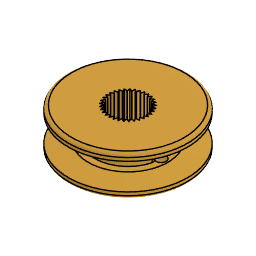
Spool_v4 (Autodesk Fusion 360 design; units mm, degrees)
Autodesk Fusion 360 part; units mm, degrees
sketch "Sketch1" plane through (0, 0, 0) normal (0, 0, 1) x (1, 0, 0)
  line L0 (-0.0246, -2.4999) -> (0.1607, -2.8207)
  line L1 (0.1607, -2.8207) -> (0.3083, -2.4809)
  arc A0 (0.3083, -2.4809) -> (0.449, -2.4594) centre (0, 0) ccw
  line L2 (0.449, -2.4594) -> (0.6916, -2.7393)
  line L3 (0.6916, -2.7393) -> (0.7722, -2.3777)
  arc A1 (0.7722, -2.3777) -> (0.9063, -2.3299) centre (0, 0) ccw
  line L4 (0.9063, -2.3299) -> (1.1975, -2.5589)
  line L5 (1.1975, -2.5589) -> (1.2083, -2.1886)
  arc A2 (1.2083, -2.1886) -> (1.3309, -2.1163) centre (0, 0) ccw
  line L6 (1.3309, -2.1163) -> (1.6601, -2.286)
  line L7 (1.6601, -2.286) -> (1.6006, -1.9204)
  arc A3 (1.6006, -1.9204) -> (1.7073, -1.8262) centre (0, 0) ccw
  line L8 (1.7073, -1.8262) -> (2.0628, -1.9306)
  line L9 (2.0628, -1.9306) -> (1.9351, -1.5828)
  arc A4 (1.9351, -1.5828) -> (2.0221, -1.4701) centre (0, 0) ccw
  line L10 (2.0221, -1.4701) -> (2.3909, -1.5053)
  line L11 (2.3909, -1.5053) -> (2.1997, -1.188)
  arc A5 (2.1997, -1.188) -> (2.2638, -1.0608) centre (0, 0) ccw
  line L12 (2.2638, -1.0608) -> (2.6325, -1.0256)
  line L13 (2.6325, -1.0256) -> (2.3848, -0.7502)
  arc A6 (2.3848, -0.7502) -> (2.4236, -0.6133) centre (0, 0) ccw
  line L14 (2.4236, -0.6133) -> (2.7791, -0.5089)
  line L15 (2.7791, -0.5089) -> (2.4837, -0.2853)
  arc A7 (2.4837, -0.2853) -> (2.4959, -0.1435) centre (0, 0) ccw
  line L16 (2.4959, -0.1435) -> (2.8251, 0.0263)
  line L17 (2.8251, 0.0263) -> (2.4928, 0.1899)
  arc A8 (2.4928, 0.1899) -> (2.4779, 0.3314) centre (0, 0) ccw
  line L18 (2.4779, 0.3314) -> (2.7691, 0.5605)
  line L19 (2.7691, 0.5605) -> (2.4118, 0.6582)
  arc A9 (2.4118, 0.6582) -> (2.3704, 0.7944) centre (0, 0) ccw
  line L20 (2.3704, 0.7944) -> (2.613, 1.0744)
  line L21 (2.613, 1.0744) -> (2.2436, 1.1028)
  arc A10 (2.2436, 1.1028) -> (2.1772, 1.2287) centre (0, 0) ccw
  line L22 (2.1772, 1.2287) -> (2.3625, 1.5495)
  line L23 (2.3625, 1.5495) -> (1.9944, 1.5074)
  arc A11 (1.9944, 1.5074) -> (1.9054, 1.6185) centre (0, 0) ccw
  line L24 (1.9054, 1.6185) -> (2.0265, 1.9686)
  line L25 (2.0265, 1.9686) -> (1.6731, 1.8576)
  arc A12 (1.6731, 1.8576) -> (1.5646, 1.9498) centre (0, 0) ccw
  line L26 (1.5646, 1.9498) -> (1.6173, 2.3165)
  line L27 (1.6173, 2.3165) -> (1.2913, 2.1407)
  arc A13 (1.2913, 2.1407) -> (1.1674, 2.2107) centre (0, 0) ccw
  line L28 (1.1674, 2.2107) -> (1.1497, 2.5807)
  line L29 (1.1497, 2.5807) -> (0.8628, 2.3464)
  arc A14 (0.8628, 2.3464) -> (0.7279, 2.3917) centre (0, 0) ccw
  line L30 (0.7279, 2.3917) -> (0.6405, 2.7517)
  line L31 (0.6405, 2.7517) -> (0.4032, 2.4673)
  arc A15 (0.4032, 2.4673) -> (0.2621, 2.4862) centre (0, 0) ccw
  line L32 (0.2621, 2.4862) -> (0.1082, 2.8232)
  line L33 (0.1082, 2.8232) -> (-0.0711, 2.499)
  arc A16 (-0.0711, 2.499) -> (-0.2132, 2.4909) centre (0, 0) ccw
  line L34 (-0.2132, 2.4909) -> (-0.4281, 2.7926)
  line L35 (-0.4281, 2.7926) -> (-0.5427, 2.4404)
  arc A17 (-0.5427, 2.4404) -> (-0.6807, 2.4055) centre (0, 0) ccw
  line L36 (-0.6807, 2.4055) -> (-0.9488, 2.6612)
  line L37 (-0.9488, 2.6612) -> (-0.9948, 2.2936)
  arc A18 (-0.9948, 2.2936) -> (-1.1237, 2.2332) centre (0, 0) ccw
  line L38 (-1.1237, 2.2332) -> (-1.4353, 2.4335)
  line L39 (-1.4353, 2.4335) -> (-1.4108, 2.0639)
  arc A19 (-1.4108, 2.0639) -> (-1.526, 1.9802) centre (0, 0) ccw
  line L40 (-1.526, 1.9802) -> (-1.8699, 2.1179)
  line L41 (-1.8699, 2.1179) -> (-1.7759, 1.7596)
  arc A20 (-1.7759, 1.7596) -> (-1.8732, 1.6556) centre (0, 0) ccw
  line L42 (-1.8732, 1.6556) -> (-2.2369, 1.7257)
  line L43 (-2.2369, 1.7257) -> (-2.0768, 1.3917)
  arc A21 (-2.0768, 1.3917) -> (-2.1527, 1.2712) centre (0, 0) ccw
  line L44 (-2.1527, 1.2712) -> (-2.5231, 1.2712)
  line L45 (-2.5231, 1.2712) -> (-2.3027, 0.9735)
  arc A22 (-2.3027, 0.9735) -> (-2.3543, 0.8409) centre (0, 0) ccw
  line L46 (-2.3543, 0.8409) -> (-2.7181, 0.7707)
  line L47 (-2.7181, 0.7707) -> (-2.4453, 0.5201)
  arc A23 (-2.4453, 0.5201) -> (-2.4709, 0.3801) centre (0, 0) ccw
  line L48 (-2.4709, 0.3801) -> (-2.8148, 0.2424)
  line L49 (-2.8148, 0.2424) -> (-2.4995, 0.0479)
  arc A24 (-2.4995, 0.0479) -> (-2.4982, -0.0944) centre (0, 0) ccw
  line L50 (-2.4982, -0.0944) -> (-2.8098, -0.2947)
  line L51 (-2.8098, -0.2947) -> (-2.4634, -0.426)
  arc A25 (-2.4634, -0.426) -> (-2.4352, -0.5655) centre (0, 0) ccw
  line L52 (-2.4352, -0.5655) -> (-2.7033, -0.8211)
  line L53 (-2.7033, -0.8211) -> (-2.3383, -0.8845)
  arc A26 (-2.3383, -0.8845) -> (-2.2842, -1.0161) centre (0, 0) ccw
  line L54 (-2.2842, -1.0161) -> (-2.499, -1.3179)
  line L55 (-2.499, -1.3179) -> (-2.1287, -1.311)
  arc A27 (-2.1287, -1.311) -> (-2.0506, -1.4301) centre (0, 0) ccw
  line L56 (-2.0506, -1.4301) -> (-2.2045, -1.767)
  line L57 (-2.2045, -1.767) -> (-1.8421, -1.6902)
  arc A28 (-1.8421, -1.6902) -> (-1.7429, -1.7923) centre (0, 0) ccw
  line L58 (-1.7429, -1.7923) -> (-1.8302, -2.1523)
  line L59 (-1.8302, -2.1523) -> (-1.4889, -2.0083)
  arc A29 (-1.4889, -2.0083) -> (-1.3722, -2.0897) centre (0, 0) ccw
  line L60 (-1.3722, -2.0897) -> (-1.3898, -2.4598)
  line L61 (-1.3898, -2.4598) -> (-1.0819, -2.2538)
  arc A30 (-1.0819, -2.2538) -> (-0.9519, -2.3117) centre (0, 0) ccw
  line L62 (-0.9519, -2.3117) -> (-0.8992, -2.6783)
  line L63 (-0.8992, -2.6783) -> (-0.6359, -2.4178)
  arc A31 (-0.6359, -2.4178) -> (-0.4972, -2.4501) centre (0, 0) ccw
  line L64 (-0.4972, -2.4501) -> (-0.3761, -2.8001)
  line L65 (-0.3761, -2.8001) -> (-0.1668, -2.4944)
  arc A32 (-0.1668, -2.4944) -> (-0.0246, -2.4999) centre (0, 0) ccw
  arc A33 (1.6969, 1.9699) -> (1.6716, 1.9914) centre (0, 0) ccw
  line L66 (1.6716, 1.9914) -> (1.7446, 2.4987)
  line L67 (1.7446, 2.4987) -> (1.2934, 2.2555)
  arc A34 (1.2934, 2.2555) -> (1.2646, 2.2718) centre (0, 0) ccw
  line L68 (1.2646, 2.2718) -> (1.2401, 2.7837)
  line L69 (1.2401, 2.7837) -> (0.8432, 2.4595)
  arc A35 (0.8432, 2.4595) -> (0.8118, 2.47) centre (0, 0) ccw
  line L70 (0.8118, 2.47) -> (0.6909, 2.9681)
  line L71 (0.6909, 2.9681) -> (0.3625, 2.5746)
  arc A36 (0.3625, 2.5746) -> (0.3296, 2.579) centre (0, 0) ccw
  line L72 (0.3296, 2.579) -> (0.1167, 3.0452)
  line L73 (0.1167, 3.0452) -> (-0.1313, 2.5967)
  arc A37 (-0.1313, 2.5967) -> (-0.1644, 2.5948) centre (0, 0) ccw
  line L74 (-0.1644, 2.5948) -> (-0.4617, 3.0123)
  line L75 (-0.4617, 3.0123) -> (-0.6204, 2.5249)
  arc A38 (-0.6204, 2.5249) -> (-0.6525, 2.5168) centre (0, 0) ccw
  line L76 (-0.6525, 2.5168) -> (-1.0235, 2.8705)
  line L77 (-1.0235, 2.8705) -> (-1.087, 2.3619)
  arc A39 (-1.087, 2.3619) -> (-1.117, 2.3478) centre (0, 0) ccw
  line L78 (-1.117, 2.3478) -> (-1.5482, 2.6249)
  line L79 (-1.5482, 2.6249) -> (-1.5143, 2.1135)
  arc A40 (-1.5143, 2.1135) -> (-1.5411, 2.094) centre (0, 0) ccw
  line L80 (-1.5411, 2.094) -> (-2.017, 2.2845)
  line L81 (-2.017, 2.2845) -> (-1.887, 1.7887)
  arc A41 (-1.887, 1.7887) -> (-1.9096, 1.7645) centre (0, 0) ccw
  line L82 (-1.9096, 1.7645) -> (-2.4129, 1.8615)
  line L83 (-2.4129, 1.8615) -> (-2.1914, 1.3993)
  arc A42 (-2.1914, 1.3993) -> (-2.209, 1.3712) centre (0, 0) ccw
  line L84 (-2.209, 1.3712) -> (-2.7216, 1.3712)
  line L85 (-2.7216, 1.3712) -> (-2.4166, 0.9593)
  arc A43 (-2.4166, 0.9593) -> (-2.4286, 0.9284) centre (0, 0) ccw
  line L86 (-2.4286, 0.9284) -> (-2.9319, 0.8313)
  line L87 (-2.9319, 0.8313) -> (-2.5544, 0.4846)
  arc A44 (-2.5544, 0.4846) -> (-2.5604, 0.452) centre (0, 0) ccw
  line L88 (-2.5604, 0.452) -> (-3.0362, 0.2615)
  line L89 (-3.0362, 0.2615) -> (-2.6, -0.0076)
  arc A45 (-2.6, -0.0076) -> (-2.5997, -0.0407) centre (0, 0) ccw
  line L90 (-2.5997, -0.0407) -> (-3.0309, -0.3179)
  line L91 (-3.0309, -0.3179) -> (-2.5516, -0.4995)
  arc A46 (-2.5516, -0.4995) -> (-2.545, -0.532) centre (0, 0) ccw
  line L92 (-2.545, -0.532) -> (-2.9159, -0.8857)
  line L93 (-2.9159, -0.8857) -> (-2.4109, -0.9734)
  arc A47 (-2.4109, -0.9734) -> (-2.3983, -1.004) centre (0, 0) ccw
  line L94 (-2.3983, -1.004) -> (-2.6956, -1.4216)
  line L95 (-2.6956, -1.4216) -> (-2.1831, -1.4121)
  arc A48 (-2.1831, -1.4121) -> (-2.165, -1.4398) centre (0, 0) ccw
  line L96 (-2.165, -1.4398) -> (-2.3779, -1.906)
  line L97 (-2.3779, -1.906) -> (-1.8764, -1.7997)
  arc A49 (-1.8764, -1.7997) -> (-1.8534, -1.8235) centre (0, 0) ccw
  line L98 (-1.8534, -1.8235) -> (-1.9742, -2.3216)
  line L99 (-1.9742, -2.3216) -> (-1.5019, -2.1223)
  arc A50 (-1.5019, -2.1223) -> (-1.4748, -2.1413) centre (0, 0) ccw
  line L100 (-1.4748, -2.1413) -> (-1.4991, -2.6532)
  line L101 (-1.4991, -2.6532) -> (-1.0731, -2.3682)
  arc A51 (-1.0731, -2.3682) -> (-1.0429, -2.3817) centre (0, 0) ccw
  line L102 (-1.0429, -2.3817) -> (-0.9699, -2.889)
  line L103 (-0.9699, -2.889) -> (-0.6056, -2.5285)
  arc A52 (-0.6056, -2.5285) -> (-0.5733, -2.536) centre (0, 0) ccw
  line L104 (-0.5733, -2.536) -> (-0.4056, -3.0204)
  line L105 (-0.4056, -3.0204) -> (-0.1161, -2.5974)
  arc A53 (-0.1161, -2.5974) -> (-0.083, -2.5987) centre (0, 0) ccw
  line L106 (-0.083, -2.5987) -> (0.1733, -3.0425)
  line L107 (0.1733, -3.0425) -> (0.3776, -2.5724)
  arc A54 (0.3776, -2.5724) -> (0.4103, -2.5674) centre (0, 0) ccw
  line L108 (0.4103, -2.5674) -> (0.746, -2.9548)
  line L109 (0.746, -2.9548) -> (0.8576, -2.4545)
  arc A55 (0.8576, -2.4545) -> (0.8888, -2.4434) centre (0, 0) ccw
  line L110 (0.8888, -2.4434) -> (1.2917, -2.7602)
  line L111 (1.2917, -2.7602) -> (1.3066, -2.2478)
  arc A56 (1.3066, -2.2478) -> (1.3351, -2.231) centre (0, 0) ccw
  line L112 (1.3351, -2.231) -> (1.7907, -2.4659)
  line L113 (1.7907, -2.4659) -> (1.7084, -1.96)
  arc A57 (1.7084, -1.96) -> (1.7332, -1.938) centre (0, 0) ccw
  line L114 (1.7332, -1.938) -> (2.225, -2.0824)
  line L115 (2.225, -2.0824) -> (2.0484, -1.6012)
  arc A58 (2.0484, -1.6012) -> (2.0687, -1.575) centre (0, 0) ccw
  line L116 (2.0687, -1.575) -> (2.5789, -1.6237)
  line L117 (2.5789, -1.6237) -> (2.3145, -1.1846)
  arc A59 (2.3145, -1.1846) -> (2.3294, -1.155) centre (0, 0) ccw
  line L118 (2.3294, -1.155) -> (2.8396, -1.1063)
  line L119 (2.8396, -1.1063) -> (2.4968, -0.7252)
  arc A60 (2.4968, -0.7252) -> (2.5059, -0.6933) centre (0, 0) ccw
  line L120 (2.5059, -0.6933) -> (2.9976, -0.5489)
  line L121 (2.9976, -0.5489) -> (2.5889, -0.2396)
  arc A61 (2.5889, -0.2396) -> (2.5918, -0.2066) centre (0, 0) ccw
  line L122 (2.5918, -0.2066) -> (3.0473, 0.0283)
  line L123 (3.0473, 0.0283) -> (2.5875, 0.2547)
  arc A62 (2.5875, 0.2547) -> (2.584, 0.2877) centre (0, 0) ccw
  line L124 (2.584, 0.2877) -> (2.9869, 0.6045)
  line L125 (2.9869, 0.6045) -> (2.4925, 0.7398)
  arc A63 (2.4925, 0.7398) -> (2.4829, 0.7715) centre (0, 0) ccw
  line L126 (2.4829, 0.7715) -> (2.8185, 1.1589)
  line L127 (2.8185, 1.1589) -> (2.3075, 1.1982)
  arc A64 (2.3075, 1.1982) -> (2.292, 1.2275) centre (0, 0) ccw
  line L128 (2.292, 1.2275) -> (2.5483, 1.6714)
  line L129 (2.5483, 1.6714) -> (2.039, 1.6132)
  arc A65 (2.039, 1.6132) -> (2.0183, 1.639) centre (0, 0) ccw
  line L130 (2.0183, 1.639) -> (2.1859, 2.1234)
  line L131 (2.1859, 2.1234) -> (1.6969, 1.9699)
  circle A66 centre (0, 0) radius 9
  circle A67 centre (0, 0) radius 5
  circle A68 centre (-5, 0) radius 0.75
  circle A69 centre (5, 0) radius 0.75
  circle A70 centre (0, 0) radius 1.7
  dimension "d1" = 0.1
  dimension "d2" = 18
  dimension "d5" = 10
  dimension "d9" = 1.5
  dimension "d10" = 1.5
  dimension "d19" = 3.4
  constraint concentric A0 A66
  constraint concentric A0 A67
  constraint coincident A67 A68.centre
  constraint coincident A67 A69.centre
  constraint concentric A66 A70
  measures "d2" diameter of A66
  measures "d5" diameter of A67
  measures "d9" diameter of A68
  measures "d10" diameter of A69
  measures "d19" diameter of A70
extrude "Extrude1" add sketch "Sketch1" along normal blind 6 contours A66 | A67 A69 | A67 A69 | A67 A68 A69 | A67 A68 | A67 A68
extrude "Extrude2" cut sketch "Sketch1" along normal blind 3 from surface at 1.5 contours A66 | A67 A69 | A67 A68 picked at (5.2368, 0.1571) picked at (-5.2458, 0)
extrude "Extrude3" cut sketch "Sketch1" along normal blind 4.5 contours A67 A69 | A67 A69 | A67 A68 | A67 A68
fillet "Fillet1" radius 0.5 4 edges at (-4.9437, -0.7479, 3) (-4.9437, 0.7479, 3) (4.9437, -0.7479, 3) (4.9437, 0.7479, 3)
fillet "Fillet2" radius 0.5 2 edges at (-8.3909, -3.2545, 0) (-8.3909, -3.2545, 6)
chamfer "Chamfer1" distance 0.5 distance2 3 2 edges at (-8.3909, 3.2545, 1.5) (-8.3909, -3.2545, 4.5) measured on face at (8.9553, -0.8961, 0.8333) measured on face at (8.9553, -0.8961, 4.8333) tangent chain off
extrude "Extrude4" add sketch "Sketch1" along normal blind 2 contours L0 L1 A0 L2 L3 A1 L4 L5 A2 L6 L7 A3 L8 L9 A4 L10 L11 A5 L12 L13 A6 L14 L15 A7 L16 L17 A8 L18 L19 A9 L20 L21 A10 L22 L23 A11 L24 L25 A12 L26 L27 A13 L28 L29 A14 L30 L31 A15 L32 L33 A16 L34 L35 A17 L36 L37 A18 L38 L39 A19 L40 L41 A20 L42 L43 A21 L44 L45 A22 L46 L47 A23 L48 L49 A24 L50 L51 A25 L52 L53 A26 L54 L55 A27 L56 L57 A28 L58 L59 A29 L60 L61 A30 L62 L63 A31 L64 L65 A32 | A33 L66 L67 A34 L68 L69 A35 L70 L71 A36 L72 L73 A37 L74 L75 A38 L76 L77 A39 L78 L79 A40 L80 L81 A41 L82 L83 A42 L84 L85 A43 L86 L87 A44 L88 L89 A45 L90 L91 A46 L92 L93 A47 L94 L95 A48 L96 L97 A49 L98 L99 A50 L100 L101 A51 L102 L103 A52 L104 L105 A53 L106 L107 A54 L108 L109 A55 L110 L111 A56 L112 L113 A57 L114 L115 A58 L116 L117 A59 L118 L119 A60 L120 L121 A61 L122 L123 A62 L124 L125 A63 L126 L127 A64 L128 L129 A65 L130 L131
fillet "Fillet3" radius 0.5 1 edges at (-1.585, 0.6147, 2)
